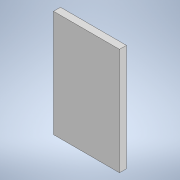
# Autodesk Inventor part: collection motor mount
Saved by Autodesk Inventor 2021 (Build 250183000, 183)
## iProperties
Created: 2021-01-07
Part Number: collection motor mount
Material: Generic
Document SubType Name: Modeling
Designer: User
Density: 1 g/cm^3
Appearance: Default
Author: User
Autodesk Inventor part; units mm, degrees
ref_plane "YZ Plane" through (0, 0, 0) normal (1, 0, 0) x (0, 1, 0)
ref_plane "XZ Plane" through (0, 0, 0) normal (0, 1, 0) x (-1, 0, 0)
ref_plane "XY Plane" through (0, 0, 0) normal (0, 0, 1) x (1, 0, 0)
sketch "Sketch1" plane through (0, 0, 0) normal (0, 0, 1) x (1, 0, 0)
  line L0 (0, 0) -> (24.13, 0)
  line L1 (24.13, 0) -> (24.13, 39.116)
  line L2 (24.13, 39.116) -> (0, 39.116)
  line L3 (0, 39.116) -> (0, 0)
  dimension "d0" = 39.116
  dimension "d1" = 24.13
  constraints: 8 end point, 2 parallel, 1 horizontal, 1 perpendicular
  measures "d0" distance of L0.end L1.end
  measures "d1" distance of L1.end L2.end
extrude "Extrusion1" add sketch "Sketch1" along normal blind 2.54
sketch "Sketch3" plane through (0, 0, 0) normal (0, -1, 0) x (1, 0, 0)
  circle A0 centre (3.9772, 1.2808) radius 0.9652
  circle A1 centre (20.3157, 1.2808) radius 0.9652
  point P0 (0, 0)
  dimension "d7" = 1.9304
  dimension "d8" = 1.9304
  constraints: 2 centre point
  measures "d7" diameter of A0
  measures "d8" diameter of A1
hole "Hole1" at (3.9772, 0, 1.2808) at (20.3157, 0, 1.2808) direction (0, 1, 0) diameter 1.6942 depth 5.7785 tip angle 118 thread size "2-56 UNC" class "2B" standard "ANSI Unified Screw Threads"
body "Solid1"
